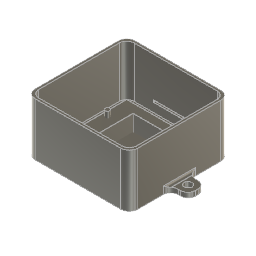
inner_camera_enclosure (Autodesk Fusion 360 design; units mm, degrees)
Autodesk Fusion 360 part; units mm, degrees
sketch "Sketch1" plane through (0, 0, 0) normal (0, 0, 1) x (1, 0, 0)
  line L0 (12.5, -12) -> (-12.5, -12)
  line L1 (-12.5, -12) -> (-12.5, 12)
  line L2 (-12.5, 12) -> (12.5, 12)
  line L3 (12.5, 12) -> (12.5, -12)
  line L4 (12.5, -12) -> (-12.5, 12) construction
  line L5 (-12.5, -12) -> (12.5, 12) construction
  line L6 (-12.5, -12) -> (-12.5, -9.5) construction
  line L7 (-12.5, -9.5) -> (-12.5, 6.4) construction
  line L8 (-12.5, -12) -> (-4.35, -12) construction
  line L9 (-4.35, -12) -> (5.75, -12) construction
  line L10 (-12.5, -12) -> (-10.6, -12) construction
  line L11 (-12.5, -12) -> (-12.5, -10.1) construction
  line L12 (-12.5, -10.1) -> (12.5, -10.1) construction
  line L13 (-10.6, -12) -> (-10.6, 12) construction
  line L14 (-12.5, 12) -> (-12.5, 10.1) construction
  line L15 (-12.5, 10.1) -> (12.5, 10.1) construction
  line L16 (12.5, 12) -> (10.6, 12) construction
  line L17 (10.6, 12) -> (10.6, -12) construction
  circle A0 centre (-10.6, 10.1) radius 1.125
  circle A1 centre (10.6, 10.1) radius 1.125
  circle A2 centre (-10.6, -10.1) radius 1.125
  circle A3 centre (10.6, -10.1) radius 1.125
  line L18 (-12.5, -9.5) -> (12.5, -9.5) construction
  line L19 (-12.5, 6.4) -> (12.5, 6.4) construction
  line L20 (-4.35, -12) -> (-4.35, 12) construction
  line L21 (5.75, -12) -> (5.75, 12) construction
  line L22 (-4.35, 6.4) -> (5.75, 6.4)
  line L23 (5.75, 6.4) -> (5.75, -9.5)
  line L24 (5.75, -9.5) -> (-4.35, -9.5)
  line L25 (-4.35, -9.5) -> (-4.35, 6.4)
  dimension "d1" = 25
  dimension "d2" = 24
  dimension "d3" = 2.5
  dimension "d4" = 15.9
  dimension "d5" = 8.15
  dimension "d6" = 10.1
  dimension "d7" = 1.9
  dimension "d8" = 1.9
  dimension "d9" = 1.9
  dimension "d10" = 1.9
  dimension "d11" = 2.25
  dimension "d12" = 2.25
  dimension "d13" = 2.25
  dimension "d14" = 2.25
  constraint horizontal L0
  constraint perpendicular L0 L1
  constraint parallel L0 L2
  constraint parallel L1 L3
  constraint coincident L4 origin
  constraint coincident L5 origin
  constraint perpendicular L0 L6
  constraint parallel L1 L7
  constraint perpendicular L1 L8
  constraint perpendicular L1 L9
  constraint perpendicular L1 L10
  constraint perpendicular L0 L11
  constraint coincident L3 L12.end
  constraint perpendicular L3 L12
  constraint coincident L2 L13.end
  constraint perpendicular L2 L13
  constraint perpendicular L2 L14
  constraint coincident L3 L15.end
  constraint perpendicular L3 L15
  constraint perpendicular L3 L16
  constraint coincident L0 L17.end
  constraint perpendicular L0 L17
  constraint coincident L13 A0.centre
  constraint coincident L15 A0.centre
  constraint coincident L15 A1.centre
  constraint coincident L17 A1.centre
  constraint coincident L13 A2.centre
  constraint coincident L12 A2.centre
  constraint coincident L12 A3.centre
  constraint coincident L17 A3.centre
  constraint coincident L3 L18.end
  constraint perpendicular L3 L18
  constraint coincident L3 L19.end
  constraint perpendicular L3 L19
  constraint coincident L2 L20.end
  constraint perpendicular L2 L20
  constraint coincident L2 L21.end
  constraint perpendicular L2 L21
  constraint coincident L19 L22.start
  constraint coincident L20 L22.start
  constraint coincident L19 L22.end
  constraint coincident L21 L22.end
  constraint coincident L18 L23.end
  constraint coincident L21 L23.end
  constraint coincident L18 L24.end
  constraint coincident L20 L24.end
  measures "d1" distance of L1.end L2.end L6
  measures "d2" distance of L0.end L1.end L6
  measures "d3" distance of L0.end L7.start L6
  measures "d4" distance of L7.start L7.end L6
  measures "d5" distance of L0.end L8.end L6
  measures "d6" distance of L8.end L9.end
  measures "d7" distance of L0.end L10.end L6
  measures "d8" distance of L0.end L11.end L6
  measures "d9" distance of L1.end L14.end L6
  measures "d10" distance of L2.end L16.end L6
  measures "d11" diameter of A0
  measures "d12" diameter of A1
  measures "d13" diameter of A2
  measures "d14" diameter of A3
sketch "Sketch2" plane through (0, 0, 0) normal (0, 0, 1) x (1, 0, 0)
  line L0 (19, -18.5) -> (-19, -18.5)
  line L1 (-19, -18.5) -> (-19, 18.5)
  line L2 (-19, 18.5) -> (19, 18.5)
  line L3 (19, 18.5) -> (19, -18.5)
  line L4 (19, -18.5) -> (-19, 18.5) construction
  line L5 (-19, -18.5) -> (19, 18.5) construction
  line L6 (19.85, -19.35) -> (-19.85, -19.35)
  line L7 (-19.85, -19.35) -> (-19.85, 19.35)
  line L8 (-19.85, 19.35) -> (19.85, 19.35)
  line L9 (19.85, 19.35) -> (19.85, -19.35)
  line L10 (19.85, -19.35) -> (-19.85, 19.35) construction
  line L11 (-19.85, -19.35) -> (19.85, 19.35) construction
  dimension "d15" = 38
  dimension "d16" = 37
  dimension "d17" = 39.7
  dimension "d18" = 38.7
  constraint horizontal L0
  constraint perpendicular L0 L1
  constraint parallel L0 L2
  constraint parallel L1 L3
  constraint coincident L4 origin
  constraint coincident L5 origin
  constraint horizontal L6
  constraint perpendicular L6 L7
  constraint parallel L6 L8
  constraint parallel L7 L9
  constraint coincident L10 origin
  constraint coincident L11 origin
  measures "d15" distance of L1.end L2.end
  measures "d16" distance of L0.end L1.end
  measures "d17" distance of L7.end L8.end
  measures "d18" distance of L6.end L7.end
extrude "Extrude1" add sketch "Sketch2" along normal blind 2 contours L0 L1 L2 L3 | L6 L7 L8 L9 makes body 1
extrude "Extrude2" add sketch "Sketch2" along normal blind 21.4 separate body makes body 2
sketch "Sketch3" plane through (0, 0, 2) normal (0, 0, 1) x (-1, 0, 0)
  line L0 (-19.85, -19.35) -> (19.85, -19.35)
  line L1 (19.85, -19.35) -> (19.85, 19.35)
  line L2 (19.85, 19.35) -> (-19.85, 19.35)
  line L3 (-19.85, 19.35) -> (-19.85, -19.35)
  circle A0 centre (10.6, -2.3) radius 1.4
  circle A1 centre (10.6, -2.3) radius 0.9
  circle A2 centre (10.6, 10.1) radius 0.9
  circle A3 centre (10.6, 10.1) radius 1.4
  circle A4 centre (-10.6, 10.1) radius 0.9
  circle A5 centre (-10.6, 10.1) radius 1.4
  circle A6 centre (-10.6, -2.3) radius 0.9
  circle A7 centre (-10.6, -2.3) radius 1.4
  dimension "d23" = 2.8
  dimension "d24" = 1.8
  dimension "d25" = 2.8
  dimension "d26" = 1.8
  dimension "d27" = 2.8
  dimension "d28" = 1.8
  dimension "d29" = 2.8
  dimension "d30" = 1.8
  constraint concentric A0 A1
  constraint concentric A2 A3
  constraint concentric A4 A5
  constraint concentric A6 A7
  measures "d23" diameter of A0
  measures "d24" diameter of A1
  measures "d25" diameter of A3
  measures "d26" diameter of A2
  measures "d27" diameter of A5
  measures "d28" diameter of A4
  measures "d29" diameter of A7
  measures "d30" diameter of A6
extrude "Extrude3" add sketch "Sketch3" along normal blind 4.7 contours A0 | A1 | A2 | A3 | A4 | A5 | A6 | A7 bodies 1
extrude "Extrude4" add sketch "Sketch3" along normal blind 7.7 separate body contours A1 | A2 | A4 | A6 makes body 3 at (9.7011, -10.0551, 7.1333) makes body 4 at (9.7011, 2.3449, 7.1333) makes body 5 at (-11.4989, -10.0551, 7.1333) makes body 6 at (-11.4989, 2.3449, 7.1333)
sketch "Sketch4" plane through (0, 19.35, 0) normal (0, 1, 0) x (-1, 0, 0)
  line L0 (-19.85, 0) -> (19.85, 0)
  line L1 (19.85, 0) -> (19.85, 21.4)
  line L2 (19.85, 21.4) -> (-19.85, 21.4)
  line L3 (-19.85, 21.4) -> (-19.85, 0)
  line L4 (-19.85, 0) -> (19.85, 0) construction
  line L5 (19.85, 0) -> (19.85, 5) construction
  line L6 (19.85, 5) -> (-19.85, 5) construction
  line L7 (-19.85, 5) -> (-19.85, 0) construction
  line L8 (0, 0) -> (0, 15) construction
  line L9 (9, 4.6) -> (-9, 4.6)
  line L10 (-9, 4.6) -> (-9, 5.4)
  line L11 (-9, 5.4) -> (9, 5.4)
  line L12 (9, 5.4) -> (9, 4.6)
  line L13 (9, 4.6) -> (-9, 5.4) construction
  line L14 (-9, 4.6) -> (9, 5.4) construction
  point P0 (0, 5)
  dimension "d35" = 5
  dimension "d36" = 0.8
  constraint horizontal L4
  constraint vertical L5
  constraint horizontal L6
  constraint vertical L7
  constraint coincident L1 L5.end
  constraint coincident L0.start L3.end
  constraint coincident L8.start origin
  constraint perpendicular L6 L8
  constraint horizontal L9
  constraint perpendicular L9 L10
  constraint parallel L9 L11
  constraint parallel L10 L12
  constraint coincident L13 P0
  constraint coincident L14 P0
  constraint midpoint L6 P0
  measures "d35" distance of L0.start L6.end
  measures "d36" distance of L9.end L10.end
extrude "Extrude5" cut sketch "Sketch4" against normal blind 2 contours L9 L10 L11 L12 bodies 2
sketch "Sketch1 (2)" plane through (0, 0, 0) normal (0, 0, 1) x (-1, 0, 0) in component "Inner wall"
  line L0 (12.5, 12) -> (7.85, 12) construction
  line L1 (7.85, 12) -> (6.35, 12) construction
  line L2 (12.5, 12) -> (-12.5, 12) construction
  line L3 (-12.5, 12) -> (-12.5, 10.5) construction
  line L4 (-12.5, 10.5) -> (12.5, 10.5) construction
  line L5 (12.5, 10.5) -> (12.5, 12) construction
  line L6 (7.85, 12) -> (-9.25, 12)
  line L7 (-9.25, 12) -> (-9.25, -9.9)
  line L8 (-9.25, -9.9) -> (7.85, -9.9)
  line L9 (7.85, -9.9) -> (7.85, 12)
  line L10 (6.35, 12) -> (6.35, -9.9) construction
  line L11 (6.35, 10.5) -> (-7.75, 10.5)
  line L12 (-7.75, 10.5) -> (-7.75, -8.4)
  line L13 (-7.75, -8.4) -> (6.35, -8.4)
  line L14 (6.35, -8.4) -> (6.35, 10.5)
  dimension "d39" = 4.65
  dimension "d40" = 1.5
  dimension "d41" = 1.5
  dimension "d42" = 17.1
  dimension "d43" = 21.9
  dimension "d44" = 14.1
  dimension "d45" = 18.9
  constraint horizontal L0
  constraint parallel L0 L1
  constraint horizontal L2
  constraint vertical L3
  constraint horizontal L4
  constraint vertical L5
  constraint horizontal L6
  constraint vertical L7
  constraint horizontal L8
  constraint vertical L9
  constraint coincident L8 L10.end
  constraint perpendicular L8 L10
  constraint horizontal L11
  constraint vertical L12
  constraint horizontal L13
  constraint vertical L14
  constraint coincident L10 L11.start
  constraint coincident L4 L11.start
  measures "d39" distance of L0.start L0.end
  measures "d40" distance of L0.end L1.end
  measures "d41" distance of L0.start L4.end
  measures "d42" distance of L0.end L6.end
  measures "d43" distance of L0.end L8.end
  measures "d44" distance of L11.start L11.end
  measures "d45" distance of L11.start L13.end
extrude "Extrude1'" add sketch "Sketch1 (2)" along normal blind 7.4 separate body makes body 7 in component "Inner wall"
sketch "Sketch2 (2)" plane through (0, 0, 7.4) normal (0, 0, 1) x (-1, 0, 0) in component "Inner wall"
  line L0 (6.35, 10.5) -> (6.35, -8.4)
  line L1 (6.35, -8.4) -> (-7.75, -8.4)
  line L2 (-7.75, -8.4) -> (-7.75, 10.5)
  line L3 (-7.75, 10.5) -> (6.35, 10.5)
  line L4 (7.85, -9.9) -> (7.85, 12)
  line L5 (7.85, 12) -> (-9.25, 12)
  line L6 (-9.25, 12) -> (-9.25, -9.9)
  line L7 (-9.25, -9.9) -> (7.85, -9.9)
  line L8 (6.35, -8.4) -> (3.85, -8.4)
  line L9 (3.85, -8.4) -> (3.85, -5.9) construction
  line L10 (3.85, -5.9) -> (6.35, -5.9) construction
  line L11 (6.35, -5.9) -> (6.35, -8.4)
  line L12 (6.35, -5.9) -> (3.85, -8.4)
  line L13 (-7.75, -8.4) -> (-5.25, -8.4)
  line L14 (-7.75, -8.4) -> (-7.75, -5.9)
  line L15 (-7.75, -5.9) -> (-5.25, -8.4)
  line L16 (6.35, 10.5) -> (3.85, 10.5)
  line L17 (6.35, 10.5) -> (6.35, 8)
  line L18 (3.85, 10.5) -> (6.35, 8)
  line L19 (-7.75, 10.5) -> (-5.25, 10.5)
  line L20 (-7.75, 10.5) -> (-7.75, 8)
  line L21 (-7.75, 8) -> (-5.25, 10.5)
  dimension "d48" = 2.5
  dimension "d49" = 2.5
  dimension "d50" = 2.5
  dimension "d51" = 2.5
  dimension "d52" = 2.5
  dimension "d53" = 2.5
  constraint horizontal L8
  constraint vertical L9
  constraint horizontal L10
  constraint vertical L11
  constraint coincident L0.end L1.start
  constraint coincident L1.end L2.start
  constraint coincident L1 L13.end
  constraint perpendicular L13 L14
  constraint coincident L0.start L3.end
  constraint perpendicular L0 L16
  constraint coincident L0 L17.end
  constraint perpendicular L16 L17
  constraint coincident L2.end L3.start
  constraint perpendicular L2 L19
  constraint coincident L2 L20.end
  constraint perpendicular L19 L20
  measures "d48" distance of L0.end L8.end
  measures "d49" distance of L0.end L10.end
  measures "d50" distance of L1.end L13.end
  measures "d51" distance of L1.end L14.end
  measures "d52" distance of L0.start L16.end
  measures "d53" distance of L2.end L19.end
sketch "Sketch3 (2)" plane through (0, 8.4, 0) normal (0, -1, 0) x (1, 0, 0) in component "Inner wall"
  line L0 (-6.35, 0) -> (7.75, 0)
  line L1 (7.75, 0) -> (7.75, 7.4)
  line L2 (7.75, 7.4) -> (-6.35, 7.4)
  line L3 (-6.35, 7.4) -> (-6.35, 0)
  line L4 (-6.35, 7.4) -> (-6.35, 4.9)
  line L5 (-6.35, 7.4) -> (-3.85, 7.4)
  line L6 (-3.85, 7.4) -> (-6.35, 4.9)
  dimension "d54" = 2.5
  dimension "d55" = 2.5
  constraint coincident L2.end L3.start
  constraint perpendicular L2 L4
  constraint perpendicular L4 L5
  measures "d54" distance of L2.end L4.end
  measures "d55" distance of L2.end L5.end
sketch "Sketch4 (2)" plane through (-6.35, 0, 0) normal (1, 0, 0) x (0, 1, 0) in component "Inner wall"
  line L0 (-10.5, 0) -> (8.4, 0)
  line L1 (8.4, 0) -> (8.4, 7.4)
  line L2 (8.4, 7.4) -> (-10.5, 7.4)
  line L3 (-10.5, 7.4) -> (-10.5, 0)
  line L4 (8.4, 7.4) -> (8.4, 4.9)
  line L5 (8.4, 7.4) -> (5.9, 7.4)
  line L6 (5.9, 7.4) -> (8.4, 4.9)
  dimension "d56" = 2.5
  constraint coincident L1.end L2.start
  constraint perpendicular L2 L4
  constraint coincident L2 L5.end
  constraint perpendicular L4 L5
  measures "d56" distance of L1.end L4.end
revolve "Revolve1" add sketch "Sketch3 (2)" angle 90 about axis through (-6.35, 8.4, 7.4) along (0, 0, -1) contours L2 L3 L4 L5 L6 bodies 7 in component "Inner wall"
sketch "Sketch5" plane through (7.75, 0, 0) normal (-1, 0, 0) x (0, -1, 0) in component "Inner wall"
  line L0 (-8.4, 0) -> (10.5, 0)
  line L1 (10.5, 0) -> (10.5, 7.4)
  line L2 (10.5, 7.4) -> (-8.4, 7.4)
  line L3 (-8.4, 7.4) -> (-8.4, 0)
  line L4 (-8.4, 7.4) -> (-5.9, 7.4)
  line L5 (-8.4, 7.4) -> (-8.4, 4.9)
  line L6 (-5.9, 7.4) -> (-8.4, 4.9)
  line L7 (10.5, 7.4) -> (8, 7.4)
  line L8 (10.5, 7.4) -> (10.5, 4.9)
  line L9 (10.5, 4.9) -> (8, 7.4)
  dimension "d58" = 2.5
  dimension "d59" = 2.5
  dimension "d60" = 2.5
  constraint coincident L2.end L3.start
  constraint perpendicular L3 L4
  constraint perpendicular L4 L5
  constraint coincident L1.end L2.start
  constraint coincident L2 L7.end
  constraint perpendicular L1 L7
  constraint perpendicular L7 L8
  measures "d58" distance of L2.end L4.end
  measures "d59" distance of L2.end L5.end
  measures "d60" distance of L1.end L8.end
revolve "Revolve2" add sketch "Sketch5" angle 90 about axis through (7.75, -10.5, 0) along (0, 0, 1) contours L1 L2 L7 L8 L9 bodies 7 in component "Inner wall"
revolve "Revolve3" add sketch "Sketch5" angle 90 about axis through (7.75, 8.4, 7.4) along (0, 0, -1) contours L2 L3 L4 L5 L6 bodies 7 in component "Inner wall"
sketch "Sketch6" plane through (-6.35, -1.05, 3.7) normal (1, 0, 0) x (0, 1, 0) in component "Inner wall"
  line L0 (-9.45, 3.7) -> (-6.95, 3.7)
  line L1 (-9.45, 3.7) -> (-9.45, 1.2)
  line L2 (-9.45, 1.2) -> (-6.95, 3.7)
  dimension "d63" = 2.5
  constraint horizontal L0
  constraint perpendicular L0 L1
  measures "d63" distance of L0.start L0.end
revolve "Revolve4" add sketch "Sketch6" angle 90 about axis through (-6.35, -10.5, 7.4) along (0, 0, -1) bodies 7 in component "Inner wall"
extrude "Extrude2'" add sketch "Sketch1 (2)" along normal blind 11.8 separate body makes body 8 in component "Inner wall"
combine "Combine1" operation add target body 1 tool bodies 5 6 2 3 4
combine "Combine1'" operation add target body 7 tool bodies 8 in component "Inner wall"
sketch "Sketch5 (2)" plane through (0, 0, 0) normal (0, 0, 1) x (1, 0, 0)
  line L0 (19, -18.5) -> (-19, -18.5)
  line L1 (-19, -18.5) -> (-19, 18.5)
  line L2 (-19, 18.5) -> (19, 18.5)
  line L3 (19, 18.5) -> (19, -18.5)
  line L4 (19, -18.5) -> (-19, 18.5) construction
  line L5 (-19, -18.5) -> (19, 18.5) construction
  line L6 (20.7, -20.2) -> (-20.7, -20.2)
  line L7 (-20.7, -20.2) -> (-20.7, 20.2)
  line L8 (-20.7, 20.2) -> (20.7, 20.2)
  line L9 (20.7, 20.2) -> (20.7, -20.2)
  line L10 (20.7, -20.2) -> (-20.7, 20.2) construction
  line L11 (-20.7, -20.2) -> (20.7, 20.2) construction
  dimension "d72" = 41.4
  dimension "d73" = 40.4
  constraint horizontal L0
  constraint perpendicular L0 L1
  constraint parallel L0 L2
  constraint parallel L1 L3
  constraint coincident L4 origin
  constraint coincident L5 origin
  constraint horizontal L6
  constraint perpendicular L6 L7
  constraint parallel L6 L8
  constraint parallel L7 L9
  constraint coincident L10 origin
  constraint coincident L11 origin
  measures "d72" distance of L7.end L8.end
  measures "d73" distance of L6.end L7.end
extrude "Extrude6" add sketch "Sketch5 (2)" along normal blind 21.4 bodies 1
sketch "Sketch6 (2)" plane through (0, 20.2, 0) normal (0, 1, 0) x (-1, 0, 0)
  line L0 (-20.7, 0) -> (20.7, 0)
  line L1 (20.7, 0) -> (20.7, 21.4)
  line L2 (20.7, 21.4) -> (-20.7, 21.4)
  line L3 (-20.7, 21.4) -> (-20.7, 0)
  line L4 (-9, 5.4) -> (9, 5.4)
  line L5 (9, 5.4) -> (9, 4.6)
  line L6 (9, 4.6) -> (-9, 4.6)
  line L7 (-9, 4.6) -> (-9, 5.4)
  constraint horizontal L4
  constraint vertical L5
  constraint horizontal L6
  constraint vertical L7
extrude "Extrude7" cut sketch "Sketch6 (2)" against normal blind 2 contours L4 L5 L6 L7 bodies 1
sketch "Sketch8" plane through (0, 0, 0) normal (0, 0, 1) x (1, 0, 0) in component "Inner wall"
  line L0 (9.25, -12) -> (9.25, -7) construction
  line L1 (9.25, -7) -> (9.25, -4) construction
  line L2 (9.25, -4) -> (13.75, -4)
  line L3 (13.75, -4) -> (13.75, -7)
  line L4 (13.75, -7) -> (9.25, -7)
  line L5 (9.25, -4) -> (9.25, -7)
  line L6 (9.25, -7) -> (-7.85, -7) construction
  line L7 (-7.85, -7) -> (-7.85, -4) construction
  line L8 (-7.85, -4) -> (9.25, -4) construction
  line L9 (9.25, -4) -> (9.25, -7) construction
  line L10 (-7.85, -7) -> (-13.75, -7)
  line L11 (-13.75, -7) -> (-13.75, -4)
  line L12 (-13.75, -4) -> (-7.85, -4)
  line L13 (-7.85, -4) -> (-7.85, -7)
  dimension "d78" = 5
  dimension "d79" = 4.5
  dimension "d80" = 5.9
  constraint vertical L0
  constraint parallel L0 L1
  constraint perpendicular L1 L2
  constraint perpendicular L2 L3
  constraint perpendicular L1 L4
  constraint horizontal L6
  constraint vertical L7
  constraint horizontal L8
  constraint vertical L9
  constraint horizontal L10
  constraint vertical L11
  constraint horizontal L12
  constraint vertical L13
  measures "d78" distance of L0.start L0.end
  measures "d79" distance of L1.end L2.end
  measures "d80" distance of L6.end L10.end
extrude "Extrude3'" add sketch "Sketch8" along normal blind 1.5 bodies 7 in component "Inner wall"
sketch "Sketch9" plane through (0, 0, 0) normal (0, 0, -1) x (1, 0, 0) in component "Inner wall"
  line L0 (-6.35, -8.4) -> (-6.35, 10.5)
  line L1 (-6.35, 10.5) -> (7.75, 10.5)
  line L2 (7.75, 10.5) -> (7.75, -8.4)
  line L3 (7.75, -8.4) -> (-6.35, -8.4)
  line L4 (-7.85, 4) -> (-7.85, -9.9)
  line L5 (-7.85, -9.9) -> (9.25, -9.9)
  line L6 (9.25, -9.9) -> (9.25, 4)
  line L7 (9.25, 4) -> (13.75, 4)
  line L8 (13.75, 4) -> (13.75, 7)
  line L9 (13.75, 7) -> (9.25, 7)
  line L10 (9.25, 7) -> (9.25, 12)
  line L11 (9.25, 12) -> (-7.85, 12)
  line L12 (-7.85, 12) -> (-7.85, 7)
  line L13 (-7.85, 7) -> (-13.75, 7)
  line L14 (-13.75, 7) -> (-13.75, 4)
  line L15 (-13.75, 4) -> (-7.85, 4)
  line L16 (-13.75, 7) -> (-12.55, 7)
  line L17 (-12.55, 7) -> (-12.55, 4)
  line L18 (-12.55, 4) -> (-13.75, 4)
  line L19 (-13.75, 4) -> (-13.75, 7)
  line L20 (13.75, 7) -> (12.55, 7)
  line L21 (12.55, 7) -> (12.55, 4)
  line L22 (12.55, 4) -> (13.75, 4)
  line L23 (13.75, 4) -> (13.75, 7)
  dimension "d83" = 1.2
  dimension "d84" = 3
  dimension "d85" = 1.2
  constraint horizontal L16
  constraint vertical L17
  constraint horizontal L18
  constraint vertical L19
  constraint coincident L13.end L14.start
  constraint horizontal L20
  constraint vertical L21
  constraint horizontal L22
  constraint vertical L23
  constraint coincident L8.end L9.start
  measures "d83" distance of L13.end L16.end
  measures "d84" distance of L13.end L14.end
  measures "d85" distance of L8.end L20.end
extrude "Extrude4'" add sketch "Sketch9" along normal blind 2 contours L13 L14 L15 L16 L17 L18 L19 | L7 L8 L9 L20 L21 L22 L23 bodies 7 in component "Inner wall"
sketch "Sketch10" plane through (12.55, 0, 0) normal (-1, 0, 0) x (0, -1, 0) in component "Inner wall"
  line L0 (7, 0) -> (4, 0)
  line L1 (4, 0) -> (4, -2)
  line L2 (4, -2) -> (7, -2)
  line L3 (7, -2) -> (7, 0)
  line L4 (7, -2) -> (4, -2) construction
  line L5 (4, -2) -> (4, 0) construction
  line L6 (4, 0) -> (7, 0) construction
  line L7 (7, 0) -> (7, -2) construction
  line L8 (7, -2) -> (4, -2)
  line L9 (4, -2) -> (4, -1)
  line L10 (4, -1) -> (7, -1)
  line L11 (7, -1) -> (7, -2)
  constraint horizontal L4
  constraint vertical L5
  constraint horizontal L6
  constraint vertical L7
  constraint coincident L0.end L1.start
  constraint coincident L2.end L3.start
  constraint horizontal L8
  constraint vertical L9
  constraint horizontal L10
  constraint vertical L11
  constraint midpoint L5 L9.end
sketch "Sketch11" plane through (0, -7, 0) normal (0, -1, 0) x (1, 0, 0) in component "Inner wall"
  line L0 (13.75, -2) -> (13.75, 1.5)
  line L1 (13.75, 1.5) -> (9.25, 1.5)
  line L2 (9.25, 1.5) -> (9.25, 0)
  line L3 (9.25, 0) -> (12.55, 0)
  line L4 (12.55, 0) -> (12.55, -2)
  line L5 (12.55, -2) -> (13.75, -2)
  line L6 (12.55, -2) -> (12.55, -1)
  line L7 (12.55, -1) -> (12.3, -1)
  line L8 (12.3, -1) -> (12.55, -2)
  line L9 (-12.55, 0) -> (-12.55, -2)
  line L10 (-12.55, -2) -> (-12.55, -1)
  line L11 (-12.55, -1) -> (-12.3, -1)
  line L12 (-12.3, -1) -> (-12.55, -2)
  constraint coincident L4.end L5.start
  constraint midpoint L4 L6.end
  constraint perpendicular L6 L7
  constraint perpendicular L5 L9
  constraint midpoint L9 L10.end
  constraint perpendicular L5 L10
  constraint perpendicular L9 L11
extrude "Extrude5'" add sketch "Sketch11" against normal blind 3 contours L4 L6 L7 L8 | L9 L10 L11 L12 bodies 7 in component "Inner wall"
extrude "Extrude6'" cut 1 faces at (-7.35, 2.1, 11.8) along direction (0, 0, -1) blind 4.4 on bodies 7 bodies 7 in component "Inner wall"
extrude "Extrude7'" cut sketch "Sketch1 (2)" along normal blind 9 contours L11 L12 L13 L14 bodies 7 in component "Inner wall"
sketch "Sketch7" plane through (0, 0, 7.4) normal (0, 0, 1) x (-1, 0, 0)
  line L0 (-7.75, -8.4) -> (-7.75, 10.5)
  line L1 (-7.75, 10.5) -> (6.35, 10.5)
  line L2 (6.35, 10.5) -> (6.35, -8.4)
  line L3 (6.35, -8.4) -> (-7.75, -8.4)
  line L4 (7.85, -9.9) -> (7.85, 12)
  line L5 (7.85, 12) -> (-9.25, 12)
  line L6 (-9.25, 12) -> (-9.25, -9.9)
  line L7 (-9.25, -9.9) -> (7.85, -9.9)
  line L8 (12.5, -12) -> (-12.5, -12)
  line L9 (-12.5, -12) -> (-12.5, 12)
  line L10 (-12.5, 12) -> (12.5, 12)
  line L11 (12.5, 12) -> (12.5, -12)
  line L12 (6.35, -8.4) -> (-7.75, -8.4)
  line L13 (-7.75, -8.4) -> (-7.75, 10.5) construction
  line L14 (-7.75, 10.5) -> (6.35, 10.5) construction
  line L15 (6.35, 10.5) -> (6.35, -8.4) construction
  line L16 (12.5, 12) -> (-12.5, 12) construction
  line L17 (-12.5, 12) -> (-12.5, 5.85) construction
  line L18 (-12.5, 5.85) -> (12.5, 5.85) construction
  line L19 (12.5, 5.85) -> (12.5, 12) construction
  line L20 (6.35, 5.85) -> (-7.75, 5.85)
  line L21 (6.35, -8.4) -> (6.35, 5.85)
  line L22 (-7.75, 5.85) -> (-7.75, -8.4)
  dimension "d94" = 6.15
  constraint horizontal L8
  constraint vertical L9
  constraint horizontal L10
  constraint vertical L11
  constraint horizontal L12
  constraint vertical L13
  constraint horizontal L14
  constraint vertical L15
  constraint coincident L0.end L1.start
  constraint coincident L2.end L3.start
  constraint horizontal L16
  constraint vertical L17
  constraint horizontal L18
  constraint vertical L19
  constraint coincident L18 L20.start
  constraint coincident L15 L20.start
  constraint coincident L18 L20.end
  constraint coincident L13 L20.end
  measures "d94" distance of L10.end L18.end
extrude "Extrude8" add sketch "Sketch7" against normal blind 1 contours L0 L1 L2 L20 | L4 L5 L6 L7 L10 | L4 L6 L7 L8 L9 L10 L11 bodies 7 in component "Inner wall"
sketch "Sketch8 (2)" plane through (0, 0, 2) normal (0, 0, 1) x (-1, 0, 0)
  line L0 (19, -18.5) -> (19, 18.5)
  line L1 (19, 18.5) -> (-19, 18.5)
  line L2 (-19, 18.5) -> (-19, -18.5)
  line L3 (-19, -18.5) -> (19, -18.5)
  circle A0 centre (10.6, 10.1) radius 1.4
  circle A1 centre (10.6, -2.3) radius 1.4
  circle A2 centre (-10.6, 10.1) radius 1.4
  circle A3 centre (-10.6, -2.3) radius 1.4
  line L4 (20.7, 0) -> (27.7, 0) construction
  line L5 (27.7, 0) -> (24.2, 0) construction
  line L6 (23.7, 3.5) -> (24.7, 3.5)
  line L7 (27.7, 0.5) -> (27.7, -0.5)
  line L8 (24.7, -3.5) -> (23.7, -3.5)
  line L9 (20.7, -3.5) -> (20.7, 3.5)
  line L10 (20.7, 3.5) -> (27.7, -3.5) construction
  line L11 (27.7, 3.5) -> (20.7, -3.5) construction
  circle A4 centre (24.2, 0) radius 1.6
  arc A5 (24.7, -3.5) -> (27.7, -0.5) centre (24.7, -0.5) ccw
  arc A6 (27.7, 0.5) -> (24.7, 3.5) centre (24.7, 0.5) ccw
  line L12 (20.7, -9.4458) -> (20.7, -6.5)
  arc A7 (23.7, -3.5) -> (20.7, -6.5) centre (23.7, -6.5) ccw
  line L13 (20.7, 2.6403) -> (20.7, 11.5)
  line L14 (20.7, 11.5) -> (20.7, 6.5)
  arc A8 (20.7, 6.5) -> (23.7, 3.5) centre (23.7, 6.5) ccw
  line L15 (-20.7, 3.5) -> (-27.7, -3.5) construction
  line L16 (-27.7, 0) -> (-24.2, 0) construction
  line L17 (-24.7, -3.5) -> (-23.7, -3.5)
  line L18 (-20.7, 0) -> (-27.7, 0) construction
  line L19 (-20.7, 11.5) -> (-20.7, 6.5)
  line L20 (-20.7, 2.6403) -> (-20.7, 11.5)
  line L21 (-27.7, 3.5) -> (-20.7, -3.5) construction
  line L22 (-20.7, -3.5) -> (-20.7, 3.5)
  line L23 (-27.7, 0.5) -> (-27.7, -0.5)
  line L24 (-23.7, 3.5) -> (-24.7, 3.5)
  arc A9 (-20.7, 6.5) -> (-23.7, 3.5) centre (-23.7, 6.5) cw
  arc A10 (-23.7, -3.5) -> (-20.7, -6.5) centre (-23.7, -6.5) cw
  arc A11 (-27.7, 0.5) -> (-24.7, 3.5) centre (-24.7, 0.5) cw
  arc A12 (-24.7, -3.5) -> (-27.7, -0.5) centre (-24.7, -0.5) cw
  circle A13 centre (-24.2, 0) radius 1.6
  line L25 (-20.7, -9.4458) -> (-20.7, -6.5)
  line L26 (20.7, -9.4458) -> (20.7, 11.5)
  line L27 (-20.7, -9.4458) -> (-20.7, 11.5)
  point P0 (24.2, 0)
  point P1 (-24.2, 0)
  dimension "d97" = 7
  dimension "d98" = 7
  dimension "d99" = 7
  dimension "d100" = 3.2
  dimension "d105" = 3
  dimension "d106" = 3
  dimension "d107" = 3
  dimension "d108" = 3
  dimension "d109" = 7
  dimension "d110" = 7
  dimension "d111" = 7
  dimension "d112" = 3.2
  dimension "d113" = 3
  dimension "d114" = 3
  dimension "d115" = 3
  dimension "d116" = 3
  constraint perpendicular L0 L4
  constraint midpoint L4 P0
  constraint horizontal L6
  constraint perpendicular L6 L7
  constraint parallel L6 L8
  constraint parallel L7 L9
  constraint coincident L10 P0
  constraint coincident L11 P0
  constraint coincident P0 L5.end
  constraint coincident L10.end L8
  constraint coincident L10.end L7
  constraint tangent L8 A5
  constraint tangent L7 A5
  constraint coincident L11.start L7
  constraint coincident L11.start L6
  constraint tangent L7 A6
  constraint tangent L6 A6
  constraint perpendicular L6 L12
  constraint coincident L9.start L8
  constraint tangent L12 A7
  constraint tangent L8 A7
  constraint coincident L9 L13.start
  constraint parallel L9 L13
  constraint perpendicular L4 L14
  constraint coincident L9.end L6
  constraint tangent L6 A8
  constraint tangent L14 A8
  constraint midpoint P1 L18
  constraint perpendicular L23 L24
  constraint parallel L17 L24
  constraint parallel L22 L23
  constraint coincident P1 L15
  constraint coincident P1 L21
  constraint coincident P1 L16.end
  constraint coincident L15.end L17
  constraint coincident L15.end L23
  constraint tangent L17 A12
  constraint tangent L23 A12
  constraint coincident L21.start L23
  constraint coincident L21.start L24
  constraint tangent L23 A11
  constraint tangent L24 A11
  constraint perpendicular L24 L25
  constraint coincident L21.end L17
  constraint tangent A10 L25
  constraint tangent L17 A10
  constraint coincident L20.start L22
  constraint parallel L20 L22
  constraint perpendicular L18 L19
  constraint coincident L15.start L24
  constraint tangent L24 A9
  constraint tangent L19 A9
  constraint parallel L13 L26
  constraint perpendicular L18 L27
  measures "d97" distance of L4.start L4.end
  measures "d98" distance of L10.end L9.start
  measures "d99" distance of L11.start L10.end
  measures "d100" diameter of A4
  measures "d105" radius of A5
  measures "d106" radius of A6
  measures "d107" radius of A7
  measures "d108" radius of A8
  measures "d109" distance of L16.start L18.start
  measures "d110" distance of L15.end L21.end
  measures "d111" distance of L15.end L21.start
  measures "d112" diameter of A13
  measures "d113" radius of A12
  measures "d114" radius of A11
  measures "d115" radius of A10
  measures "d116" radius of A9
extrude "Extrude8'" add sketch "Sketch8 (2)" against normal blind 2 contours L6 L7 L8 L9 A5 A6 A7 L13 A8 L26 | L17 L20 L22 L23 L24 A9 A10 A11 A12 L27 bodies 1
extrude "Extrude9" cut 1 faces at (-3.3, 13.5041, 2) along direction (0, 0, -1) blind 1 on bodies 1 bodies 1
sketch "Sketch9 (2)" plane through (0, 0, 1) normal (0, 0, 1) x (-1, 0, 0)
  line L0 (19, -18.5) -> (19, 18.5)
  line L1 (19, 18.5) -> (-19, 18.5)
  line L2 (-19, 18.5) -> (-19, -18.5)
  line L3 (-19, -18.5) -> (19, -18.5)
  circle A0 centre (10.6, 10.1) radius 1.4
  circle A1 centre (10.6, -2.3) radius 1.4
  circle A2 centre (-10.6, 10.1) radius 1.4
  circle A3 centre (-10.6, -2.3) radius 1.4
  line L4 (-19.7, 19.2) -> (19.7, 19.2)
  line L5 (19.7, 19.2) -> (19.7, -19.2)
  line L6 (19.7, -19.2) -> (-19.7, -19.2)
  line L7 (-19.7, -19.2) -> (-19.7, 19.2)
  line L8 (-19.7, 19.2) -> (19.7, -19.2) construction
  line L9 (19.7, 19.2) -> (-19.7, -19.2) construction
  line L10 (19, -18.5) -> (-19, -18.5)
  line L11 (-19, -18.5) -> (-19, 18.5)
  line L12 (-19, 18.5) -> (19, 18.5)
  line L13 (19, 18.5) -> (19, -18.5)
  dimension "d121" = 39.4
  dimension "d122" = 38.4
  constraint horizontal L4
  constraint perpendicular L4 L5
  constraint parallel L4 L6
  constraint parallel L5 L7
  constraint coincident L8 origin
  constraint coincident L9 origin
  constraint horizontal L10
  constraint vertical L11
  constraint horizontal L12
  constraint vertical L13
  constraint coincident L1.end L2.start
  constraint coincident L0.start L3.end
  measures "d121" distance of L5.end L6.end
  measures "d122" distance of L4.end L5.end
extrude "Extrude10" cut sketch "Sketch9 (2)" along normal blind 22 contours L4 L5 L6 L7 bodies 1
fillet "Fillet1" radius 1 1 edges at (20.7, 0, 2) on bodies 1
fillet "Fillet2" radius 1 1 edges at (-20.7, 0, 2) on bodies 1
fillet "Fillet3" radius 3 1 edges at (-19.7, 19.2, 11.2) on bodies 1
fillet "Fillet4" radius 3.5 1 edges at (-20.7, 20.2, 10.7) on bodies 1
fillet "Fillet5" radius 3 1 edges at (19.7, 19.2, 11.2) on bodies 1
fillet "Fillet6" radius 3 1 edges at (19.7, -19.2, 11.2) on bodies 1
fillet "Fillet7" radius 3 1 edges at (-19.7, -19.2, 11.2) on bodies 1
fillet "Fillet8" radius 3.5 1 edges at (20.7, 20.2, 10.7) on bodies 1
fillet "Fillet9" radius 3.5 1 edges at (20.7, -20.2, 10.7) on bodies 1
fillet "Fillet10" radius 3.5 1 edges at (-20.7, -20.2, 10.7) on bodies 1
component "Inner wall" placed x (1, 0, 0) y (0, 1, 0) z (0, 0, 1) at (0, 0, 0)
